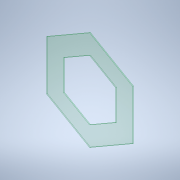
# Autodesk Inventor part: Membrane
Saved by Autodesk Inventor 2020.3 (Build 243373000, 373)
## iProperties
Created: 2020-07-07
Part Number: Membrane
Material: Nylon 6/6
Document SubType Name: Modeling
Designer: Bruno
Density: 1.13 g/cm^3
Appearance: Clear - Green 1
Author: Bruno
Autodesk Inventor part; units mm, degrees
ref_plane "YZ Plane" through (0, 0, 0) normal (1, 0, 0) x (0, 1, 0)
ref_plane "XZ Plane" through (0, 0, 0) normal (0, 1, 0) x (-1, 0, 0)
ref_plane "Work Plane1" through (0, 0, 0) normal (0, 0, 1) x (1, 0, 0)
sketch "Sketch1" plane through (0, 0, 0) normal (0, 0, 1) x (1, 0, 0)
  line L0 (302, -174.3598) -> (0, -348.7196)
  line L1 (0, -348.7196) -> (-302, -174.3598)
  line L2 (-302, -174.3598) -> (-302, 174.3598)
  line L3 (-302, 174.3598) -> (0, 348.7196)
  line L4 (0, 348.7196) -> (302, 174.3598)
  line L5 (302, 174.3598) -> (302, -174.3598)
  line L6 (498, -287.5204) -> (0, -575.0409)
  line L7 (0, -575.0409) -> (-498, -287.5204)
  line L8 (-498, -287.5204) -> (-498, 287.5204)
  line L9 (-498, 287.5204) -> (0, 575.0409)
  line L10 (0, 575.0409) -> (498, 287.5204)
  line L11 (498, 287.5204) -> (498, -287.5204)
  point P0 (0, 0)
  point P1 (0, 0)
  point P2 (0, 0)
  dimension "d0" = 302
  dimension "d1" = 498
  constraints: 24 end point, 2 coincident, 2 vertical, 26 other
  measures "d0" distance from line of point (0, 0) L5
  measures "d1" distance from line of point (0, 0) L11
extrude "Extrusion1" add sketch "Sketch1" along normal blind 10
body "Solid1"
